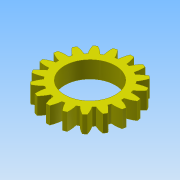
# Autodesk Inventor part: Stirnzahnrad1
Saved by Autodesk Inventor 2015 (Build 190159000, 159)
## iProperties
Created: 2015-09-09
Part Number: Stirnzahnrad1
Material: ABS-Kunststoff
Document SubType Name: Modeling
Designer: Johann
Categories: <?xml version="1.0" encoding="UTF-16"?> <MemberInstance><Categories><FamilyTemplate><FamilyTemplateParameter ValueType="xs:double" Id="1" ObjectReferenceKey="da_z" ObjectType="kUserParameterObject"/><FamilyTemplateParameter ValueType="xs:double" Id="2" ObjectReferenceKey="da_b" ObjectType="kUserParameterObject"/><FamilyTemplateParameter ValueType="xs:double" Id="3" ObjectReferenceKey="da_beta" ObjectType="kUserParameterObject"/><FamilyTemplateParameter ValueType="xs:double" Id="4" ObjectReferenceKey="da_da" ObjectType="kUserParameterObject"/><FamilyTemplateParameter ValueType="xs:double" Id="5" ObjectReferenceKey="da_aw" ObjectType="kUserParameterObject"/><FamilyTemplateParameter ValueType="xs:string" Id="6" ObjectReferenceKey="EAIAABAAAACIAQAAAAAAAIAAAAAAAAAA" ObjectType="83910656" SubObjectId="SurfaceGeometry"/></FamilyTemplate><ParamToTemplateMap><ParamToTemplate CategoryParameter="//CategoryParameter[@InternalName='046C89C9-8512-4d59-83FE-43B91F4F132A']" TemplateParameter="1"/><ParamToTemplate CategoryParameter="//CategoryParameter[@InternalName='2552DF32-E462-4b46-AEBF-C6C7768E72AC']" TemplateParameter="2"/><ParamToTemplate CategoryParameter="//CategoryParameter[@InternalName='C9EE641D-15FC-4fae-A226-E94C4372FDD7']" TemplateParameter="3"/><ParamToTemplate><ParamToTemplate CategoryParameter="//CategoryParameter[@InternalName='00B6519A-459B-49c7-AD84-2E56D39A5744']" ConstantValue="0.000000"/></ParamToTemplate><ParamToTemplate><ParamToTemplate CategoryParameter="//CategoryParameter[@InternalName='04B31F0E-C7A6-4894-AA32-9629BEFACF47']" ConstantValue="1.000000"/></ParamToTemplate><ParamToTemplate><ParamToTemplate CategoryParameter="//CategoryParameter[@InternalName='43CBEC2E-7847-49e7-A936-2F7889FCB2D9']" ConstantValue="0.250000"/></ParamToTemplate><ParamToTemplate><ParamToTemplate CategoryParameter="//CategoryParameter[@InternalName='B1EFC894-105D-4ebd-86BF-FA20ED196853']" ConstantValue="0.350000"/></ParamToTemplate><ParamToTemplate><ParamToTemplate CategoryParameter="//CategoryParameter[@InternalName='51175063-3D10-4879-93E8-6246FE8B403D']" ConstantValue="2060000000.000000"/></ParamToTemplate><ParamToTemplate><ParamToTemplate CategoryParameter="//CategoryParameter[@InternalName='A3A52E27-4454-46a9-B0BD-C932399B70AF']" ConstantValue="0.300000"/></ParamToTemplate><ParamToTemplate><ParamToTemplate CategoryParameter="//CategoryParameter[@InternalName='91B76062-C214-41d9-B1B9-14D2AB99603D']" ConstantValue="0.100000"/></ParamToTemplate><ParamToTemplate><ParamToTemplate CategoryParameter="//CategoryParameter[@InternalName='374E806E-8B8A-4dda-A9AA-1039D6500AD2']" ConstantValue="10.000000"/></ParamToTemplate><ParamToTemplate><ParamToTemplate CategoryParameter="//CategoryParameter[@InternalName='2D373A89-B862-43d6-8D0B-0CBF12AB9F6C']" ConstantValue="0.349066"/></ParamToTemplate><ParamToTemplate CategoryParameter="//CategoryParameter[@InternalName='37777632-D6A2-4fac-9D53-DB8ACD95C989']" TemplateParameter="4"/><ParamToTemplate CategoryParameter="//CategoryParameter[@InternalName='FD1017F1-B727-4f7e-9707-0F86F1FF9423']" TemplateParameter="5"/><ParamToTemplate><ParamToTemplate CategoryParameter="//CategoryParameter[@InternalName='9E1B4470-B2D3-4ff1-B813-535BB4CDF51A']" ConstantValue="3520000.000000"/></ParamToTemplate><ParamToTemplate><ParamToTemplate CategoryParameter="//CategoryParameter[@InternalName='F8452263-BFF6-458c-9FB1-07C4B99E95CD']" ConstantValue="11400000.000000"/></ParamToTemplate><ParamToTemplate><ParamToTemplate CategoryParameter="//CategoryParameter[@InternalName='3E3BB259-FD49-497f-8171-6EBC954A3479']" ConstantValue="2.000000"/></ParamToTemplate><ParamToTemplate CategoryParameter="//CategoryParameter[@InternalName='27C3BAF2-7550-4e4b-AE2C-0DB134B7D9B7']" TemplateParameter="6"/></ParamToTemplateMap><Category DisplayName="Gear" InternalName="DC85795E-93AB-48d5-8EEE-5A27447B64BD" Mnemonic="Gear"><CategoryParameter DisplayName="z" InternalName="046C89C9-8512-4d59-83FE-43B91F4F132A" Mnemonic="z"/><CategoryParameter DisplayName="b" InternalName="2552DF32-E462-4b46-AEBF-C6C7768E72AC" Mnemonic="b"/><CategoryParameter DisplayName="||b|" InternalName="C9EE641D-15FC-4fae-A226-E94C4372FDD7" Mnemonic="beta"/><CategoryParameter DisplayName="x" InternalName="00B6519A-459B-49c7-AD84-2E56D39A5744" Mnemonic="x"/><CategoryParameter DisplayName="a*" InternalName="04B31F0E-C7A6-4894-AA32-9629BEFACF47" Mnemonic="a"/><CategoryParameter DisplayName="c*" InternalName="43CBEC2E-7847-49e7-A936-2F7889FCB2D9" Mnemonic="c"/><CategoryParameter DisplayName="r|.f|*" InternalName="B1EFC894-105D-4ebd-86BF-FA20ED196853" Mnemonic="rf"/><CategoryParameter DisplayName="E" InternalName="51175063-3D10-4879-93E8-6246FE8B403D" Mnemonic="E"/><CategoryParameter DisplayName="||m|" InternalName="A3A52E27-4454-46a9-B0BD-C932399B70AF" Mnemonic="mi"/><Category DisplayName="SpurGear" InternalName="26C5A22E-A91E-4dfd-A3B3-23CCAFAE1764" Mnemonic="SpurGear"><CategoryParameter DisplayName="m" InternalName="91B76062-C214-41d9-B1B9-14D2AB99603D" Mnemonic="m"/><CategoryParameter DisplayName="P" InternalName="374E806E-8B8A-4dda-A9AA-1039D6500AD2" Mnemonic="PP"/><CategoryParameter DisplayName="||a|" InternalName="2D373A89-B862-43d6-8D0B-0CBF12AB9F6C" Mnemonic="alpha"/><CategoryParameter DisplayName="d|.a|" InternalName="37777632-D6A2-4fac-9D53-DB8ACD95C989" Mnemonic="da"/><CategoryParameter DisplayName="a|.w|" InternalName="FD1017F1-B727-4f7e-9707-0F86F1FF9423" Mnemonic="aw"/><CategoryParameter DisplayName="||s||.Flim|" InternalName="9E1B4470-B2D3-4ff1-B813-535BB4CDF51A" Mnemonic="sFlim"/><CategoryParameter DisplayName="||s||.Hlim|" InternalName="F8452263-BFF6-458c-9FB1-07C4B99E95CD" Mnemonic="sHlim"/><CategoryParameter DisplayName="Typ" InternalName="3E3BB259-FD49-497f-8171-6EBC954A3479" Mnemonic="type"/><CategoryParameter DisplayName="PitchDiameter" InternalName="27C3BAF2-7550-4e4b-AE2C-0DB134B7D9B7" Mnemonic="IDS_PITCHDIAM"/></Category></Category></Categories></MemberInstance>
Density: 1.06 g/cm^3
Appearance: Glatt - gelb
Mass: 0.59095 g
Surface Area: 8.84752 cm^2
Volume: 0.5575 cm^3
CustomPartVersion: 1
Author: Johann
Autodesk Inventor part; units mm, degrees
sketch "Sketch1" plane through (0, 0, 0) normal (0, 0, 1) x (1, 0, 0)
  circle A0 centre (0, 0) radius 10
  dimension "d0" = 20
  constraints: 1 centre point
  measures "d0" diameter of A0
extrude "Extrusion1" add sketch "Sketch1" along normal blind 4
ref_plane "Work Plane2" through (0, 0, 2) normal (0, 0, 1) x (1, 0, 0)
sketch "Sketch2" plane through (0, 0, 0) normal (0, 0, -1) x (-1, 0, 0)
  circle A0 centre (0, 0) radius 10 projected
  circle A1 centre (0, 0) radius 9
  dimension "d3" = 18
  constraints: 1 centre point, 1 coincident
  measures "d3" diameter of A1
surface extrude "Flankendurchmesser" sketch "Sketch2" against normal through all shown no curves A1
ref_plane "Work Plane8" through (0, 0, 0) normal (0.9848078, 0.1736482, 0) x (0, 0, 1)
ref_plane "Work Plane9" through (0, 0, 0) normal (1, 0, 0) x (0, 1, 0)
spur gear teeth "Stirnzahnrad" teeth 18 pitch diameter 18 tip diameter 20 root diameter 15.5 face width 4 start plane through (0, 0, 0) normal (0, 0, -1) x (-1, 0, 0)
sketch "Skizze3" plane through (0, 0, 4) normal (0, 0, 1) x (1, 0, 0)
  arc A0 (-8.8701, 4.6175) -> (-7.1601, 2.9658) centre (-2.6305, 9.3664) ccw construction
  arc A1 (-7.1601, 2.9658) -> (-7.3913, 2.3305) centre (0, 0) ccw construction
  arc A2 (-7.3913, 2.3305) -> (-9.763, 2.1644) centre (-8.0357, -5.4842) ccw construction
  arc A3 (-9.763, 2.1644) -> (-9.9144, 1.3053) centre (0, 0) ccw construction
  arc A4 (-9.9144, 1.3053) -> (-7.7426, 0.3381) centre (-5.6754, 7.9019) ccw construction
  arc A5 (-7.7426, 0.3381) -> (-7.7426, -0.3381) centre (0, 0) ccw construction
  arc A6 (-7.7426, -0.3381) -> (-9.9144, -1.3053) centre (-5.6754, -7.9019) ccw construction
  arc A7 (-9.9144, -1.3053) -> (-9.763, -2.1644) centre (0, 0) ccw construction
  arc A8 (-9.763, -2.1644) -> (-7.3913, -2.3305) centre (-8.0357, 5.4842) ccw construction
  arc A9 (-7.3913, -2.3305) -> (-7.1601, -2.9658) centre (0, 0) ccw construction
  arc A10 (-7.1601, -2.9658) -> (-8.8701, -4.6175) centre (-2.6305, -9.3664) ccw construction
  arc A11 (-8.8701, -4.6175) -> (-8.4339, -5.373) centre (0, 0) ccw construction
  arc A12 (-8.4339, -5.373) -> (-6.1485, -4.7179) centre (-9.4268, 2.4051) ccw construction
  arc A13 (-6.1485, -4.7179) -> (-5.7139, -5.2358) centre (0, 0) ccw construction
  arc A14 (-5.7139, -5.2358) -> (-6.7559, -7.3728) centre (0.7316, -9.7013) ccw construction
  arc A15 (-6.7559, -7.3728) -> (-6.0876, -7.9335) centre (0, 0) ccw construction
  arc A16 (-6.0876, -7.9335) -> (-4.1641, -6.5363) centre (-9.6809, -0.9641) ccw construction
  arc A17 (-4.1641, -6.5363) -> (-3.5786, -6.8743) centre (0, 0) ccw construction
  arc A18 (-3.5786, -6.8743) -> (-3.8268, -9.2388) centre (4.0055, -8.866) ccw construction
  arc A19 (-3.8268, -9.2388) -> (-3.0071, -9.5372) centre (0, 0) ccw construction
  arc A20 (-3.0071, -9.5372) -> (-1.6774, -7.5663) centre (-8.7674, -4.217) ccw construction
  arc A21 (-1.6774, -7.5663) -> (-1.0116, -7.6837) centre (0, 0) ccw construction
  arc A22 (-1.0116, -7.6837) -> (-0.4362, -9.9905) centre (6.7963, -6.9613) ccw construction
  arc A23 (-0.4362, -9.9905) -> (0.4362, -9.9905) centre (0, 0) ccw construction
  arc A24 (0.4362, -9.9905) -> (1.0116, -7.6837) centre (-6.7963, -6.9613) ccw construction
  arc A25 (1.0116, -7.6837) -> (1.6774, -7.5663) centre (0, 0) ccw construction
  arc A26 (1.6774, -7.5663) -> (3.0071, -9.5372) centre (8.7674, -4.217) ccw construction
  arc A27 (3.0071, -9.5372) -> (3.8268, -9.2388) centre (0, 0) ccw construction
  arc A28 (3.8268, -9.2388) -> (3.5786, -6.8743) centre (-4.0055, -8.866) ccw construction
  arc A29 (3.5786, -6.8743) -> (4.1641, -6.5363) centre (0, 0) ccw construction
  arc A30 (4.1641, -6.5363) -> (6.0876, -7.9335) centre (9.6809, -0.9641) ccw construction
  arc A31 (6.0876, -7.9335) -> (6.7559, -7.3728) centre (0, 0) ccw construction
  arc A32 (6.7559, -7.3728) -> (5.7139, -5.2358) centre (-0.7316, -9.7013) ccw construction
  arc A33 (5.7139, -5.2358) -> (6.1485, -4.7179) centre (0, 0) ccw construction
  arc A34 (6.1485, -4.7179) -> (8.4339, -5.373) centre (9.4268, 2.4051) ccw construction
  arc A35 (8.4339, -5.373) -> (8.8701, -4.6175) centre (0, 0) ccw construction
  arc A36 (8.8701, -4.6175) -> (7.1601, -2.9658) centre (2.6305, -9.3664) ccw construction
  arc A37 (7.1601, -2.9658) -> (7.3913, -2.3305) centre (0, 0) ccw construction
  arc A38 (7.3913, -2.3305) -> (9.763, -2.1644) centre (8.0357, 5.4842) ccw construction
  arc A39 (9.763, -2.1644) -> (9.9144, -1.3053) centre (0, 0) ccw construction
  arc A40 (9.9144, -1.3053) -> (7.7426, -0.3381) centre (5.6754, -7.9019) ccw construction
  arc A41 (7.7426, -0.3381) -> (7.7426, 0.3381) centre (0, 0) ccw construction
  arc A42 (7.7426, 0.3381) -> (9.9144, 1.3053) centre (5.6754, 7.9019) ccw construction
  arc A43 (9.9144, 1.3053) -> (9.763, 2.1644) centre (0, 0) ccw construction
  arc A44 (9.763, 2.1644) -> (7.3913, 2.3305) centre (8.0357, -5.4842) ccw construction
  arc A45 (7.3913, 2.3305) -> (7.1601, 2.9658) centre (0, 0) ccw construction
  arc A46 (7.1601, 2.9658) -> (8.8701, 4.6175) centre (2.6305, 9.3664) ccw construction
  arc A47 (8.8701, 4.6175) -> (8.4339, 5.373) centre (0, 0) ccw construction
  arc A48 (8.4339, 5.373) -> (6.1485, 4.7179) centre (9.4268, -2.4051) ccw construction
  arc A49 (6.1485, 4.7179) -> (5.7139, 5.2358) centre (0, 0) ccw construction
  arc A50 (5.7139, 5.2358) -> (6.7559, 7.3728) centre (-0.7316, 9.7013) ccw construction
  arc A51 (6.7559, 7.3728) -> (6.0876, 7.9335) centre (0, 0) ccw construction
  arc A52 (6.0876, 7.9335) -> (4.1641, 6.5363) centre (9.6809, 0.9641) ccw construction
  arc A53 (4.1641, 6.5363) -> (3.5786, 6.8743) centre (0, 0) ccw construction
  arc A54 (3.5786, 6.8743) -> (3.8268, 9.2388) centre (-4.0055, 8.866) ccw construction
  arc A55 (3.8268, 9.2388) -> (3.0071, 9.5372) centre (0, 0) ccw construction
  arc A56 (3.0071, 9.5372) -> (1.6774, 7.5663) centre (8.7674, 4.217) ccw construction
  arc A57 (1.6774, 7.5663) -> (1.0116, 7.6837) centre (0, 0) ccw construction
  arc A58 (1.0116, 7.6837) -> (0.4362, 9.9905) centre (-6.7963, 6.9613) ccw construction
  arc A59 (0.4362, 9.9905) -> (-0.4362, 9.9905) centre (0, 0) ccw construction
  arc A60 (-0.4362, 9.9905) -> (-1.0116, 7.6837) centre (6.7963, 6.9613) ccw construction
  arc A61 (-1.0116, 7.6837) -> (-1.6774, 7.5663) centre (0, 0) ccw construction
  arc A62 (-1.6774, 7.5663) -> (-3.0071, 9.5372) centre (-8.7674, 4.217) ccw construction
  arc A63 (-3.8268, 9.2388) -> (-3.5786, 6.8743) centre (4.0055, 8.866) ccw projected
  arc A64 (-3.5786, 6.8743) -> (-4.1641, 6.5363) centre (0, 0) ccw projected
  arc A65 (-4.1641, 6.5363) -> (-6.0876, 7.9335) centre (-9.6809, 0.9641) ccw projected
  arc A66 (-6.0876, 7.9335) -> (-6.7559, 7.3728) centre (0, 0) ccw projected
  arc A67 (-6.7559, 7.3728) -> (-5.7139, 5.2358) centre (0.7316, 9.7013) ccw projected
  arc A68 (-5.7139, 5.2358) -> (-6.1485, 4.7179) centre (0, 0) ccw projected
  arc A69 (-6.1485, 4.7179) -> (-8.4339, 5.373) centre (-9.4268, -2.4051) ccw projected
  arc A70 (-8.4339, 5.373) -> (-8.8701, 4.6175) centre (0, 0) ccw projected
  arc A71 (-3.0071, 9.5372) -> (-3.8268, 9.2388) centre (0, 0) ccw projected
hole "Bohrung1" at (0, 0, 4) direction (0, 0, -1) diameter 12 end through all
equation "\"d0\" = da_da"
equation "\"d1\" = da_b"
equation "\"d3\" = da_dw"
equation "\"d16\" = da_aw"
equation "\"d43\" = da_aw"
equation "\"d46\" = da_aw"
equation "\"da_da\" = 20"
equation "\"da_b\" = 4"
equation "\"da_dw\" = 18"
equation "\"da_aw\" = 18"
body "Solid1"
body "Srf1"
